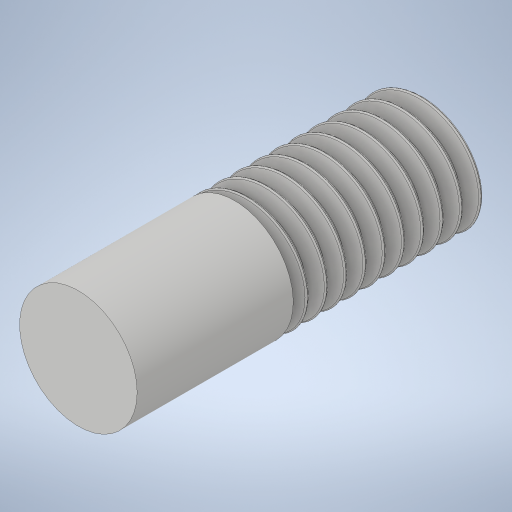
# Autodesk Inventor part: SCREW_nogap
Saved by Autodesk Inventor 2023 (Build 270158000, 158)
## iProperties
Created: 2019-05-31
Part Number: SCREW_nogap
Material: Generic
Document SubType Name: Modeling
Designer: rbarrett
Density: 1 g/cm^3
Appearance: Default
Author: rbarrett
Autodesk Inventor part; units mm, degrees
ref_plane "YZ Plane" through (0, 0, 0) normal (1, 0, 0) x (0, 1, 0)
ref_plane "XZ Plane" through (0, 0, 0) normal (0, 1, 0) x (-1, 0, 0)
ref_plane "XY Plane" through (0, 0, 0) normal (0, 0, 1) x (1, 0, 0)
sketch "Sketch1" plane through (0, 0, 0) normal (0, 0, 1) x (1, 0, 0)
  circle A0 centre (0, 0) radius 3.05
  dimension "d0" = 6.1
  constraints: 1 centre point, 1 coincident
  measures "d0" diameter of A0
extrude "Extrusion1" add sketch "Sketch1" along normal blind 18.1
thread "Thread1" size "M7x1" class "6g" standard "ANSI Metric M Profile" length 10
sketch "Sketch3" plane through (0, 0, 0) normal (1, 0, 0) x (0, 1, 0)
  line L0 (3.05, 0) -> (3.05, 10)
  line L1 (3.05, 10) -> (2.3085, 10)
  line L2 (2.3085, 10) -> (2.3085, 0)
  line L3 (2.3085, 0) -> (3.05, 0)
  line L4 (0, -4.9286) -> (0, 21.9381) projected
  constraints: 8 end point
revolve "Revolution1" cut sketch "Sketch3" angle 360 about axis through (0, 0, 0) along (0, 0, 1)
sketch "Sketch4" plane through (0, 0, 0) normal (1, 0, 0) x (0, 1, 0)
  line L0 (3.05, 0) -> (3.05, 10)
  line L1 (3.05, 10) -> (2.3085, 10)
  line L2 (2.3085, 10) -> (2.3085, 0)
  line L3 (2.3085, 0) -> (3.05, 0)
  line L4 (0, -4.9286) -> (0, 21.9381) projected
  constraints: 8 end point
revolve "Revolution2" add sketch "Sketch4" angle 360 about axis through (0, 0, 0) along (0, 0, 1) separate body
sketch "Sketch2" plane through (0, 0, 0) normal (-1, 0, 0) x (0, 0, 1)
  line L0 (-0.5834, -2.3593) -> (-0.5001, -2.3593) construction
  line L1 (0.0832, -2.9996) -> (-0.0001, -3.1597) construction
  line L2 (-1.0001, -3.1597) -> (-1.0834, -2.9996) construction
  line L3 (-0.4168, -2.3593) -> (-0.5001, -2.1992) construction
  line L4 (-0.5001, -2.1992) -> (-0.5834, -2.3593) construction
  line L5 (-1.0001, -3.1597) -> (-0.9168, -2.9996) construction
  line L6 (-0.4168, -2.3593) -> (-0.0834, -2.9996)
  line L7 (-1.0834, -2.9996) -> (-0.9168, -2.9996) construction
  arc A0 (-1.0834, -2.9996) -> (-1.0001, -3.0502) centre (-1.0001, -2.9562) ccw construction
  line L8 (0.0832, -2.9996) -> (-0.0834, -2.9996) construction
  line L9 (-1.0001, -3.1597) -> (-1.0001, -2.9996) construction
  line L10 (-0.0001, -3.1597) -> (-0.0001, -2.9996) construction
  line L11 (-0.5001, -2.1992) -> (-0.5001, -2.3087) construction
  line L12 (-1.0001, -3.0502) -> (-0.0001, -3.0502)
  arc A1 (-1.0001, -3.0502) -> (-0.9168, -2.9996) centre (-1.0001, -2.9562) ccw
  line L13 (-0.0834, -2.9996) -> (-0.0001, -3.1597) construction
  line L14 (-0.9168, -2.9996) -> (-0.5834, -2.3593)
  line L15 (-0.0001, -0.0002) -> (-0.0001, 0.0177)
  line L16 (-0.0001, 0.0177) -> (-0.0001, -0.0002)
  line L17 (-0.0001, -0.0002) -> (0.0334, -0.0002)
  arc A2 (-0.0834, -2.9996) -> (-0.0001, -3.0502) centre (-0.0001, -2.9562) ccw
  arc A3 (-0.0001, -3.0502) -> (0.0832, -2.9996) centre (-0.0001, -2.9562) ccw construction
  arc A4 (-0.5001, -2.3087) -> (-0.5834, -2.3593) centre (-0.5001, -2.4027) ccw
  arc A5 (-0.4168, -2.3593) -> (-0.5001, -2.3087) centre (-0.5001, -2.4027) ccw
  line L18 (-0.5001, -2.3087) -> (-0.5001, -2.3593) construction
  line L19 (-0.5001, -2.3593) -> (-0.4168, -2.3593) construction
  dimension "d5" = 55
  dimension "d6" = 0.1601
  dimension "d7" = 0.1601
  dimension "Sketch2_ThreadOffset" = 0
  dimension "Sketch2_MajorRadius" = 3.05
  dimension "d10" = 1
  dimension "Sketch2_MinorRadius" = 2.3085
  constraints: 40 end point, 12 point on circle, 10 parallel, 8 tangent, 6 centre point, 6 collinear, 2 midpoint, 2 point on line, 1 horizontal, 1 perpendicular, 3 other
  measures "d5" angle of L6 L14
  measures "d6" distance of L3.end L0.end
  measures "d7" distance of L1.end L10.end
  measures "Sketch2_ThreadOffset" distance between parallel lines of L15 L10
  measures "Sketch2_MajorRadius" distance from line of L12 L15.start
  measures "d10" distance from line of L1.end L9
  measures "Sketch2_MinorRadius" distance edge to line of A5 L17
coil "Coil1" sketch "Sketch2" operation cut axis through (0, 0, 0) along (0, 0, 1) pitch 1.001 turns 11.988012 hand right bodies 2
combine bodies "Combine1" operation type add bodies to combine 2 1
equation "\"d5\" = d12"
equation "\"d6\" = 0.160083 * Sketch2_Pitch"
equation "\"d7\" = 0.160083 * Sketch2_Pitch"
equation "\"d10\" = Sketch2_Pitch"
equation "\"d12\" = 55deg"
equation "\"Sketch2_Pitch\" = 1"
body "Solid1"
